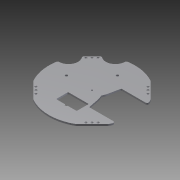
# Autodesk Inventor part: Deck
Saved by Autodesk Inventor 2011 (Build 150239000, 239)
## iProperties
Created: 2011-01-27
Part Number: Deck
Document SubType Name: Modeling
Designer: Physics Student
Density: 1 g/cm^3
Author: Physics Student
Autodesk Inventor part; units mm, degrees
ref_plane "YZ Plane" through (0, 0, 0) normal (1, 0, 0) x (0, 1, 0)
ref_plane "XZ Plane" through (0, 0, 0) normal (0, 1, 0) x (-1, 0, 0)
ref_plane "XY Plane" through (0, 0, 0) normal (0, 0, 1) x (1, 0, 0)
sketch "Sketch1" plane through (0, 0, 0) normal (0, 0, 1) x (1, 0, 0)
  circle A0 centre (0, 0) radius 171.45
  dimension "d0" = 342.9
  constraints: 1 centre point, 1 coincident
  measures "d0" diameter of A0
extrude "Extrusion1" add sketch "Sketch1" along normal blind 6.35
sketch "Sketch2" plane through (0, 0, 6.35) normal (0, 0, 1) x (1, 0, 0)
  circle A0 centre (0, 0) radius 171.45 projected
  line L0 (197.6462, 0) -> (-281.2915, 0)
  line L1 (0, -189.9673) -> (0, 254.2486)
  line L2 (0, 0) -> (-224.0806, 224.0806)
  line L3 (-117.1025, 117.1025) -> (25.0798, 259.2849)
  line L4 (25.0798, 259.2849) -> (-193.4238, 635.0058)
  line L5 (-193.4238, 635.0058) -> (-427.1769, 145.6409)
  line L6 (-427.1769, 145.6409) -> (-369.1953, -134.9902)
  line L7 (-369.1953, -134.9902) -> (-88.5642, 145.6409)
  dimension "d3" = 45
  dimension "d4" = 165.608
  constraints: 16 end point, 2 perpendicular, 2 point on line, 1 horizontal
  measures "d3" angle of L0 L2
  measures "d4" distance from line of L2.start L3
extrude "Extrusion2" cut sketch "Sketch2" against normal blind 40 contours L3 L2 A0 | A0 L7 L6 L5 L4 L3 | L7 A0 L2
pattern_circular "Circular Pattern1" count 4 over 360 about axis through (0, 0, -10) along (0, 0, 1) of "Extrusion2"
sketch "Sketch3" plane through (0, 0, 6.35) normal (0, 0, 1) x (1, 0, 0)
  arc A0 (148.48, -85.7251) -> (148.48, 85.7251) centre (0, 0) ccw projected
  circle A1 centre (0, 0) radius 3.0226
  dimension "d10" = 6.0452
  constraints: 1 centre point, 1 coincident
  measures "d10" diameter of A1
extrude "Extrusion3" cut sketch "Sketch3" against normal blind 40
sketch "Sketch4" plane through (0, 0, 6.35) normal (0, 0, 1) x (1, 0, 0)
  circle A0 centre (0, 0) radius 3.0226 projected
  circle A1 centre (-163.83, 70.358) radius 38.1
  circle A2 centre (-70.358, 163.83) radius 38.1
  dimension "d13" = 76.2
  dimension "d14" = 76.2
  dimension "d15" = 70.358
  dimension "d16" = 70.358
  dimension "d17" = 163.83
  dimension "d18" = 163.83
  constraints: 2 centre point
  measures "d13" diameter of A1
  measures "d14" diameter of A2
  measures "d15" horizontal distance of A0.centre A2.centre
  measures "d16" vertical distance of A0.centre A1.centre
  measures "d17" horizontal distance of A0.centre A1.centre
  measures "d18" vertical distance of A0.centre A2.centre
extrude "Extrusion4" cut sketch "Sketch4" against normal blind 40 contours A1 | A2
fillet "Fillet1" radius 6.35 1 edges at (-136.8978, 97.3073, 3.175)
fillet "Fillet2" radius 6.35 1 edges at (-168.3366, 32.5255, 3.175)
fillet "Fillet3" radius 6.35 1 edges at (-97.3073, 136.8978, 3.175)
fillet "Fillet4" radius 6.35 1 edges at (-32.5255, 168.3366, 3.175)
sketch "Sketch5" plane through (0, 0, 6.35) normal (0, 0, 1) x (1, 0, 0)
  arc A0 (-169.3248, 26.9115) -> (-148.48, -85.7251) centre (0, 0) ccw projected
  circle A1 centre (0, 101.6) radius 4.9022
  dimension "d25" = 9.8044
  dimension "d26" = 101.6
  constraints: 1 centre point
  measures "d25" diameter of A1
  measures "d26" distance of A0.centre A1.centre
extrude "Extrusion5" cut sketch "Sketch5" against normal blind 40
pattern_circular "Circular Pattern2" count 4 over 360 about axis through (0, 0, -10) along (0, 0, 1) of "Extrusion5"
sketch "Sketch6" plane through (0, 0, 6.35) normal (0, 0, 1) x (1, 0, 0)
  arc A0 (-169.3248, 26.9115) -> (-148.48, -85.7251) centre (0, 0) ccw projected
  circle A1 centre (0, 0) radius 3.0226 projected
  circle A2 centre (-99.4768, 123.952) radius 2.159
  line L0 (0, 0) -> (-213.9537, 213.9537)
  circle A3 centre (0, 0) radius 3.0226 projected
  line L1 (0, 0) -> (0, 193.7824)
  line L2 (-75.5206, 147.9082) -> (-146.0285, 77.4003)
  circle A4 centre (-111.7144, 111.7144) radius 2.159
  circle A5 centre (-123.952, 99.4768) radius 2.159
  line L3 (0, 0) -> (-99.4768, 123.952)
  line L4 (0, 0) -> (-123.952, 99.4768)
  dimension "d32" = 4.318
  dimension "d33" = 45
  dimension "d34" = 157.988
  dimension "d35" = 0
  dimension "d36" = 4.318
  dimension "d37" = 4.318
  dimension "d49" = 123.952
  constraints: 10 end point, 3 centre point, 3 point on line, 1 perpendicular, 1 vertical, 1 other
  measures "d32" diameter of A2
  measures "d33" angle of L1 L0
  measures "d34" distance from line of A0.centre L2
  measures "d35" distance from line of L2 L3.end
  measures "d36" diameter of A4
  measures "d37" diameter of A5
  measures "d49" vertical distance of A0.centre L3.end
extrude "Extrusion6" cut sketch "Sketch6" against normal blind 40 contours L4 L2 A5 | A5 L2 L4 | L3 L2 A2 | A2 L2 L3 | A4 L2 L0 | L0 L2 A4 | A5 L2 | A2 L2 | L2 A4 L0 | L0 A4 L2
sketch "Sketch7" plane through (0, 0, 6.35) normal (0, 0, 1) x (1, 0, 0)
  circle A0 centre (-111.7144, 111.7144) radius 2.159 projected
  circle A1 centre (-99.4768, 123.952) radius 2.159 projected
  circle A2 centre (-123.952, 99.4768) radius 2.159 projected
  circle A3 centre (-99.4768, 123.952) radius 4.2164
  circle A4 centre (-111.7144, 111.7144) radius 4.2164
  circle A5 centre (-123.952, 99.4768) radius 4.2164
  dimension "d41" = 8.4328
  dimension "d42" = 8.4328
  dimension "d43" = 8.4328
  constraints: 3 centre point, 3 coincident
  measures "d41" diameter of A3
  measures "d42" diameter of A4
  measures "d43" diameter of A5
extrude "Extrusion7" cut sketch "Sketch7" against normal blind 2.54
pattern_circular "Circular Pattern3" count 4 over 360 about axis through (0, 0, -10) along (0, 0, 1) of "Extrusion6", "Extrusion7"
sketch "Sketch13" plane through (0, 0, 6.35) normal (0, 0, 1) x (1, 0, 0)
  circle A0 centre (101.6, 0) radius 4.9022 projected
  circle A1 centre (0, 0) radius 3.0226 projected
  line L0 (220.5677, -64) -> (53, -64)
  line L1 (53, -64) -> (53, 64)
  line L2 (53, 64) -> (220.5677, 64)
  line L3 (220.5677, 64) -> (220.5677, -64)
  line L4 (0, 0) -> (36.6997, 0) construction
  line L5 (0, 0) -> (0, -29.3606) construction
  line L6 (53, 64) -> (43, 14.6803)
  line L7 (43, 14.6803) -> (37, 0)
  line L8 (53, -64) -> (43, -14.6803)
  line L9 (43, -14.6803) -> (37, 0)
  arc A2 (148.48, -85.7251) -> (148.48, 85.7251) centre (0, 0) ccw projected
  dimension "d81" = 128
  dimension "d87" = 10
  dimension "d88" = 16
  dimension "d89" = 37
  constraints: 20 end point, 3 perpendicular, 2 parallel, 1 horizontal, 1 point on line, 1 symmetric about line, 1 other
  measures "d81" distance of L2.end L0.start
  measures "d87" distance from line of L1 L6.end
  measures "d88" distance from line of L1 L7.end
  measures "d89" distance of A2.centre L7.end
extrude "Extrusion11" cut sketch "Sketch13" against normal through all contours L0 A2 L2 L3 | L0 L1 L2 A2 | L8 L9 L7 L6 L1
fillet "Fillet7" radius 40 2 edges at (43, 14.6803, 3.175) (43, -14.6803, 3.175)
fillet "Fillet8" radius 3 2 edges at (53, -64, 3.175) (53, 64, 3.175)
sketch "Sketch14" plane through (0, 0, 6.35) normal (0, 0, 1) x (1, 0, 0)
  arc A0 (159.0569, 64) -> (148.48, 85.7251) centre (0, 0) ccw projected
  circle A1 centre (0, 0) radius 3.0226 projected
  line L0 (41, -102) -> (-41, -102)
  line L1 (-41, -102) -> (-41, -54)
  line L2 (-41, -54) -> (41, -54)
  line L3 (41, -54) -> (41, -102)
  line L4 (0, 0) -> (0, -193.6891)
  dimension "d90" = 82
  dimension "d91" = 48
  dimension "d92" = 54
  constraints: 10 end point, 3 parallel, 1 horizontal, 1 perpendicular, 1 other
  measures "d90" distance of L1.end L2.end
  measures "d91" distance of L0.end L1.end
  measures "d92" distance from line of L2 A0.centre
extrude "Extrusion12" cut sketch "Sketch14" against normal blind 20 contours L2 L3 L0 L4 | L4 L0 L1 L2
fillet "Fillet9" radius 3 1 edges at (37, 0, 3.175)
fillet "Fillet10" radius 3 4 edges at (-41, -54, 3.175) (41, -54, 3.175) (41, -102, 3.175) (-41, -102, 3.175)
fillet "Fillet11" radius 2 2 edges at (4.8859, -102, 3.175) (-4.8859, -102, 3.175)
fillet "Fillet12" radius 6.5 2 edges at (159.0569, -64, 3.175) (159.0569, 64, 3.175)
body "Solid1"
